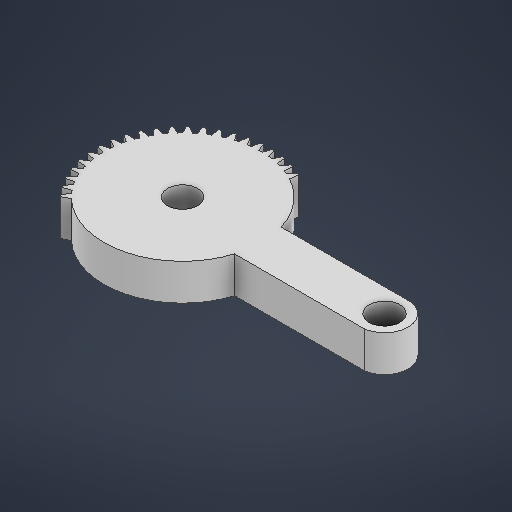
# Autodesk Inventor part: innerGear
Saved by Autodesk Inventor 2026.2 (Build 302298000, 298)
## iProperties
Created: 2026-04-07
Part Number: innerGear
Material: Generic
Document SubType Name: Modeling
Designer: Brian Wang
Density: 1 g/cm^3
Appearance: Default
Author: Brian Wang
Autodesk Inventor part; units mm, degrees
ref_plane "YZ Plane" through (0, 0, 0) normal (1, 0, 0) x (0, 1, 0)
ref_plane "XZ Plane" through (0, 0, 0) normal (0, 1, 0) x (-1, 0, 0)
ref_plane "XY Plane" through (0, 0, 0) normal (0, 0, 1) x (1, 0, 0)
sketch "Sketch1" plane through (0, 0, 0) normal (0, 1, 0) x (-1, 0, 0)
  circle A0 centre (0, 0) radius 11
  line L0 (0, 0) -> (21.5969, 0.9429) construction
  line L1 (0, 0) -> (22.384, -0.9773) construction
  line L2 (0, 0) -> (25.2479, 0) construction
  line L3 (10.9895, 0.4798) -> (12.0415, 0.1582)
  line L4 (10.9895, 0.4798) -> (12.0895, 0.4798) construction
  line L5 (10.9895, -0.4798) -> (12.0415, -0.1582)
  line L6 (12.0415, -0.1582) -> (12.0415, 0.1582)
  line L7 (10.9561, 0.9815) -> (11.9561, 1.4397)
  line L8 (11.9561, 1.4397) -> (11.9142, 1.7533)
  line L9 (10.8289, 1.9326) -> (11.9142, 1.7533)
  line L10 (10.7293, 2.4254) -> (11.6597, 3.0122)
  line L11 (11.6597, 3.0122) -> (11.5765, 3.3175)
  line L12 (10.4771, 3.3513) -> (11.5765, 3.3175)
  line L13 (10.313, 3.8266) -> (11.1574, 4.5315)
  line L14 (11.1574, 4.5315) -> (11.0345, 4.8231)
  line L15 (9.9402, 4.7109) -> (11.0345, 4.8231)
  line L16 (9.7146, 5.1602) -> (10.4581, 5.9708)
  line L17 (10.4581, 5.9708) -> (10.2976, 6.2435)
  line L18 (9.2279, 5.9872) -> (10.2976, 6.2435)
  line L19 (8.9446, 6.4026) -> (9.5741, 7.3047)
  line L20 (9.5741, 7.3047) -> (9.3789, 7.5537)
  line L21 (8.3526, 7.1578) -> (9.3789, 7.5537)
  line L22 (8.0168, 7.532) -> (8.521, 8.5096)
  line L23 (8.521, 8.5096) -> (8.2945, 8.7306)
  line L24 (7.3298, 8.2021) -> (8.2945, 8.7306)
  line L25 (6.9474, 8.5284) -> (7.3176, 9.5643)
  line L26 (7.3176, 9.5643) -> (7.0638, 9.7532)
  line L27 (6.1776, 9.1015) -> (7.0638, 9.7532)
  line L28 (5.7553, 9.3743) -> (5.9849, 10.45)
  line L29 (5.9849, 10.45) -> (5.7083, 10.6037)
  line L30 (4.9164, 9.8402) -> (5.7083, 10.6037)
  line L31 (4.4616, 10.0546) -> (4.5465, 11.1513)
  line L32 (4.5465, 11.1513) -> (4.252, 11.2669)
  line L33 (3.5683, 10.4052) -> (4.252, 11.2669)
  line L34 (3.0891, 10.5573) -> (3.0279, 11.6556)
  line L35 (3.0279, 11.6556) -> (2.7206, 11.7312)
  line L36 (2.1572, 10.7864) -> (2.7206, 11.7312)
  line L37 (1.6621, 10.8737) -> (1.4558, 11.9542)
  line L38 (1.4558, 11.9542) -> (1.1412, 11.9883)
  line L39 (0.708, 10.9772) -> (1.1412, 11.9883)
  line L40 (0.2057, 10.9981) -> (-0.142, 12.0417)
  line L41 (-0.142, 12.0417) -> (-0.4584, 12.0338)
  line L42 (-0.7536, 10.9742) -> (-0.4584, 12.0338)
  line L43 (-1.2543, 10.9283) -> (-1.7373, 11.9165)
  line L44 (-1.7373, 11.9165) -> (-2.0498, 11.8668)
  line L45 (-2.202, 10.7773) -> (-2.0498, 11.8668)
  line L46 (-2.6922, 10.6655) -> (-3.302, 11.581)
  line L47 (-3.302, 11.581) -> (-3.6051, 11.4902)
  line L48 (-3.6115, 10.3902) -> (-3.6051, 11.4902)
  line L49 (-4.0825, 10.2144) -> (-4.8083, 11.0409)
  line L50 (-4.8083, 11.0409) -> (-5.0967, 10.9108)
  line L51 (-4.9572, 9.8197) -> (-5.0967, 10.9108)
  line L52 (-5.4007, 9.5829) -> (-6.2297, 10.3059)
  line L53 (-6.2297, 10.3059) -> (-6.4983, 10.1387)
  line L54 (-6.2154, 9.0757) -> (-6.4983, 10.1387)
  line L55 (-6.6236, 8.7822) -> (-7.5411, 9.389)
  line L56 (-7.5411, 9.389) -> (-7.7852, 9.1876)
  line L57 (-7.3638, 8.1715) -> (-7.7852, 9.1876)
  line L58 (-7.7295, 7.8265) -> (-8.7194, 8.3062)
  line L59 (-8.7194, 8.3062) -> (-8.9346, 8.0743)
  line L60 (-8.3823, 7.1231) -> (-8.9346, 8.0743)
  line L61 (-8.699, 6.7326) -> (-9.7437, 7.0768)
  line L62 (-9.7437, 7.0768) -> (-9.9263, 6.8184)
  line L63 (-9.2527, 5.9488) -> (-9.9263, 6.8184)
  line L64 (-9.5148, 5.5198) -> (-10.596, 5.7225)
  line L65 (-10.596, 5.7225) -> (-10.7427, 5.4421)
  line L66 (-9.9597, 4.6695) -> (-10.7427, 5.4421)
  line L67 (-10.1627, 4.2095) -> (-11.2612, 4.2671)
  line L68 (-11.2612, 4.2671) -> (-11.3694, 3.9698)
  line L69 (-10.4909, 3.3078) -> (-11.3694, 3.9698)
  line L70 (18.6565, 53.6502) -> (-47.4327, 53.6502)
  line L71 (18.6565, 53.6502) -> (84.7457, 53.6502) construction
  line L72 (-2.4093, 65.0508) -> (-2.2907, 63.9572)
  line L73 (-2.2907, 63.9572) -> (-1.9799, 63.8978)
  line L74 (-1.4667, 64.8708) -> (-1.9799, 63.8978)
  line L75 (-0.9861, 64.8115) -> (-0.7236, 63.7432)
  line L76 (-0.7236, 63.7432) -> (-0.4077, 63.7256)
  line L77 (-0.028, 64.758) -> (-0.4077, 63.7256)
  line L78 (0.4561, 64.7629) -> (0.858, 63.739)
  line L79 (0.858, 63.739) -> (1.1734, 63.7634)
  line L80 (1.4129, 64.837) -> (1.1734, 63.7634)
  line L81 (2.4261, 63.9444) -> (2.7355, 64.0104)
  line L82 (1.892, 64.9061) -> (2.4261, 63.9444)
  line L83 (2.8305, 65.1063) -> (2.7355, 64.0104)
  line L84 (3.2962, 65.2383) -> (3.953, 64.3559)
  line L85 (3.953, 64.3559) -> (4.251, 64.4624)
  line L86 (4.1998, 65.5612) -> (4.251, 64.4624)
  line L87 (4.6438, 65.7537) -> (5.4119, 64.9662)
  line L88 (5.4119, 64.9662) -> (5.6931, 65.1113)
  line L89 (5.4967, 66.1936) -> (5.6931, 65.1113)
  line L90 (5.9112, 66.4432) -> (6.7768, 65.7645)
  line L91 (6.7768, 65.7645) -> (7.0363, 65.9456)
  line L92 (6.6982, 66.9923) -> (7.0363, 65.9456)
  line L93 (7.0759, 67.2947) -> (8.0239, 66.7367)
  line L94 (8.0239, 66.7367) -> (8.2571, 66.9506)
  line L95 (7.7831, 67.9432) -> (8.2571, 66.9506)
  line L96 (-4.2364, 65.6602) -> (-4.9873, 64.8564)
  line L97 (-2.8778, 65.1733) -> (-3.5155, 64.277)
  line L98 (-3.8157, 64.377) -> (-3.5155, 64.277)
  line L99 (-3.7882, 65.4767) -> (-3.8157, 64.377)
  line L100 (-4.2364, 65.6602) -> (-4.7195, 64.672) construction
  line L101 (-5.2716, 64.9954) -> (-4.9873, 64.8564)
  line L102 (-5.0986, 66.0817) -> (-5.2716, 64.9954)
  line L103 (8.1173, 68.2929) -> (9.1309, 67.8656)
  line L104 (9.1309, 67.8656) -> (9.3337, 68.1085)
  line L105 (8.7324, 69.0296) -> (9.3337, 68.1085)
  line L106 (10.0785, 69.1313) -> (10.2473, 69.3989)
  line L107 (9.5291, 70.2321) -> (10.2473, 69.3989)
  line L108 (9.0172, 69.4204) -> (10.0785, 69.1313)
  line L109 (9.7596, 70.6572) -> (10.8499, 70.5113)
  line L110 (10.8499, 70.5113) -> (10.9817, 70.7989)
  line L111 (10.1594, 71.5296) -> (10.9817, 70.7989)
  line L112 (10.3315, 71.9814) -> (11.4315, 71.9814)
  line L113 (11.4315, 71.9814) -> (11.524, 72.2839)
  line L114 (10.6121, 72.8991) -> (11.524, 72.2839)
  line L115 (10.7227, 73.3697) -> (11.813, 73.5155)
  line L116 (11.813, 73.5155) -> (11.8645, 73.8276)
  line L117 (10.8791, 74.3165) -> (11.8645, 73.8276)
  line L118 (10.9263, 74.7975) -> (11.9877, 75.0865)
  line L119 (11.9877, 75.0865) -> (11.9974, 75.4028)
  line L120 (10.9559, 75.7566) -> (11.9974, 75.4028)
  line L121 (10.9389, 76.2396) -> (11.9526, 76.6668)
  line L122 (11.9526, 76.6668) -> (11.9203, 76.9816)
  line L123 (10.841, 77.1942) -> (11.9203, 76.9816)
  line L124 (10.7602, 77.6706) -> (11.7083, 78.2285)
  line L125 (11.7083, 78.2285) -> (11.6345, 78.5362)
  line L126 (10.5366, 78.6038) -> (11.6345, 78.5362)
  line L127 (10.3934, 79.0652) -> (11.2591, 79.7438)
  line L128 (11.2591, 79.7438) -> (11.1452, 80.039)
  line L129 (10.048, 79.9605) -> (11.1452, 80.039)
  line L130 (9.8449, 80.3988) -> (10.613, 81.1862)
  line L131 (10.613, 81.1862) -> (10.461, 81.4637)
  line L132 (9.3839, 81.2404) -> (10.461, 81.4637)
  line L133 (9.1245, 81.6478) -> (9.7814, 82.5301)
  line L134 (9.7814, 82.5301) -> (9.5939, 82.785)
  line L135 (8.5559, 82.4209) -> (9.5939, 82.785)
  line L136 (8.2449, 82.7902) -> (8.779, 83.7518)
  line L137 (8.779, 83.7518) -> (8.5594, 83.9796)
  line L138 (7.5789, 83.4811) -> (8.5594, 83.9796)
  circle A1 centre (-27.7353, 75.6145) radius 2.125
  arc A2 (-28.2533, 78.823) -> (-28.265, 72.408) centre (-27.7353, 75.6145) ccw
  line L139 (-28.265, 72.408) -> (-10.2739, 72.408)
  line L140 (-28.2533, 78.823) -> (-10.2623, 78.823)
  circle A3 centre (0.1033, 75.6173) radius 2.075
  arc A4 (7.5789, 83.4811) -> (-10.2623, 78.823) centre (0.1033, 75.6173) ccw
  arc A5 (8.5559, 82.4209) -> (8.2449, 82.7902) centre (0.1033, 75.6173) ccw
  arc A6 (9.3839, 81.2404) -> (9.1245, 81.6478) centre (0.1033, 75.6173) ccw
  arc A7 (10.048, 79.9605) -> (9.8449, 80.3988) centre (0.1033, 75.6173) ccw
  arc A8 (10.5366, 78.6038) -> (10.3934, 79.0652) centre (0.1033, 75.6173) ccw
  arc A9 (10.841, 77.1942) -> (10.7602, 77.6706) centre (0.1033, 75.6173) ccw
  arc A10 (10.9559, 75.7566) -> (10.9389, 76.2396) centre (0.1033, 75.6173) ccw
  arc A11 (10.8791, 74.3165) -> (10.9263, 74.7975) centre (0.1033, 75.6173) ccw
  arc A12 (10.6121, 72.8991) -> (10.7227, 73.3697) centre (0.1033, 75.6173) ccw
  arc A13 (10.1594, 71.5296) -> (10.3315, 71.9814) centre (0.1033, 75.6173) ccw
  arc A14 (9.5291, 70.2321) -> (9.7596, 70.6572) centre (0.1033, 75.6173) ccw
  arc A15 (8.7324, 69.0296) -> (9.0172, 69.4204) centre (0.1033, 75.6173) ccw
  arc A16 (7.7831, 67.9432) -> (8.1173, 68.2929) centre (0.1033, 75.6173) ccw
  arc A17 (6.6982, 66.9923) -> (7.0759, 67.2947) centre (0.1033, 75.6173) ccw
  arc A18 (5.4967, 66.1936) -> (5.9112, 66.4432) centre (0.1033, 75.6173) ccw
  arc A19 (4.1998, 65.5612) -> (4.6438, 65.7537) centre (0.1033, 75.6173) ccw
  arc A20 (2.8305, 65.1063) -> (3.2962, 65.2383) centre (0.1033, 75.6173) ccw
  arc A21 (1.4129, 64.837) -> (1.892, 64.9061) centre (0.1033, 75.6173) ccw
  arc A22 (-0.028, 64.758) -> (0.4561, 64.7629) centre (0.1033, 75.6173) ccw
  arc A23 (-1.4667, 64.8708) -> (-0.9861, 64.8115) centre (0.1033, 75.6173) ccw
  arc A24 (-2.8778, 65.1733) -> (-2.4093, 65.0508) centre (0.1033, 75.6173) ccw
  arc A25 (-10.2739, 72.408) -> (-5.0986, 66.0817) centre (0.1033, 75.6173) ccw
  arc A26 (-4.2364, 65.6602) -> (-3.7882, 65.4767) centre (0.1033, 75.6173) ccw
  dimension "d0" = 22
  dimension "d1" = 2.5
  dimension "d2" = 2.5
  dimension "d3" = 1.1
  dimension "d4" = 17
  dimension "d5" = 0.3164
  dimension "d8" = 160
  dimension "d15" = 4.15
  dimension "d21" = 10.85
  constraints: 282 end point, 48 point on circle, 45 point on line, 26 centre point, 4 coincident, 3 horizontal, 2 equal length, 2 symmetric about line, 1 vertical, 172 other
  measures "d1" angle of L2 L0
  measures "d2" angle of L1 L2
  measures "d3" distance of L3.start L3.end
  measures "d4" angle of L3 L4
  measures "d5" distance of L5.end L6.end
  measures "d15" diameter of A3
  measures "d21" radius of A4
extrude "Extrusion1" add sketch "Sketch1" along normal blind 5 contours A24 L97 L98 L99 A26 L96 L101 L102 A25 L139 A2 L140 A4 L138 L137 L136 A5 L135 L134 L133 A6 L132 L131 L130 A7 L129 L128 L127 A8 L126 L125 L124 A9 L123 L122 L121 A10 L120 L119 L118 A11 L117 L116 L115 A12 L114 L113 L112 A13 L111 L110 L109 A14 L107 L106 L108 A15 L105 L104 L103 A16 L95 L94 L93 A17 L92 L91 L90 A18 L89 L88 L87 A19 L86 L85 L84 A20 L83 L81 L82 A21 L80 L79 L78 A22 L77 L76 L75 A23 L74 L73 L72
body "Solid1"
